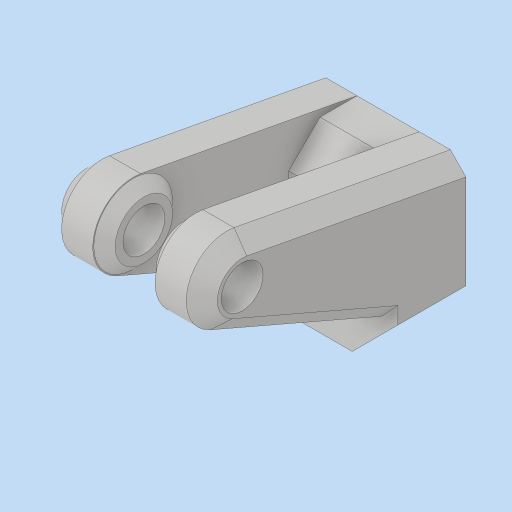
# Autodesk Inventor part: Profil-WheelHold-wBearing
Saved by Autodesk Inventor 2024 (Build 280153000, 153)
## iProperties
Created: 2023-04-19
Part Number: Profil-WheelHold-wBearing
Material: Generic
Document SubType Name: Modeling
Designer: Karbosch
Density: 1 g/cm^3
Appearance: Default
Mass: 3.2214 g
Surface Area: 21.1129 cm^2
Volume: 3.2214 cm^3
Author: Karbosch
Autodesk Inventor part; units mm, degrees
ref_plane "YZ Plane" through (0, 0, 0) normal (1, 0, 0) x (0, 1, 0)
ref_plane "XZ Plane" through (0, 0, 0) normal (0, 1, 0) x (-1, 0, 0)
ref_plane "XY Plane" through (0, 0, 0) normal (0, 0, 1) x (1, 0, 0)
sketch "Sketch1" plane through (0, 0, 0) normal (0, 0, 1) x (1, 0, 0)
  circle A0 centre (0, 0) radius 2.15
  line L0 (3.3137, 8) -> (8, 3.3137)
  line L1 (8, 3.3137) -> (8, -3.3137)
  line L2 (8, -3.3137) -> (3.3137, -8)
  line L3 (3.3137, -8) -> (-3.3137, -8)
  line L4 (-3.3137, -8) -> (-8, -3.3137)
  line L5 (-8, -3.3137) -> (-8, 3.3137)
  line L6 (-8, 3.3137) -> (-3.3137, 8)
  line L7 (-3.3137, 8) -> (3.3137, 8)
  dimension "d0" = 4.3
  dimension "d1" = 16
  constraints: 16 end point, 2 coincident, 1 centre point, 1 horizontal, 17 other
  measures "d0" diameter of A0
  measures "d1" distance between parallel lines of L3 L7
extrude "Extrusion1" add sketch "Sketch1" along normal blind 7
sketch "Sketch2" plane through (8, -3.3137, 0) normal (1, 0, 0) x (0, 0, -1)
  line L0 (0, 0) -> (-7, 0) projected
  line L1 (0, 6.6274) -> (0, 0) projected
  line L2 (0, 11.3137) -> (0, 6.6274) projected
  circle A0 centre (-23, 11.4137) radius 2.15
  circle A1 centre (-23, 11.4137) radius 4.15
  line L3 (0, 11.3137) -> (-7, 11.3137) projected
  line L4 (0, 11.3137) -> (-22.2335, 15.4923)
  line L5 (-7, 0) -> (-7, -4.6863) projected
  line L6 (-7, 0) -> (-24.6423, 7.6025)
  line L7 (-7, 1.1637) -> (-7, 5.4637) projected
  line L8 (-7, 3.3137) -> (-11, 3.3137)
  line L9 (-11, 3.3137) -> (-11, 7.0137)
  circle A2 centre (-23, 11.4137) radius 11
  circle A3 centre (-23, 11.4137) radius 8.1
  line L10 (5.8437, 3.3137) -> (-35.0625, 3.3137) projected
  point P0 (0, 3.3137)
  dimension "d4" = 4.3
  dimension "d6" = 2
  dimension "d17" = 4
  dimension "d18" = 3.7
  dimension "d19" = 22
  dimension "d33" = 16.2
  dimension "d34" = 16
  constraints: 8 end point, 4 centre point, 3 coincident, 3 tangent, 2 point on circle, 1 horizontal, 1 midpoint, 1 vertical
  measures "d4" diameter of A0
  measures "d6" radial gap between concentric circles of A1 A0
  measures "d17" distance of L8.start L8.end
  measures "d18" distance of L8.end L9.end
  measures "d19" diameter of A2
  measures "d33" diameter of A3
  measures "d34" horizontal distance of L3.end A0.centre
extrude "Extrusion2" add sketch "Sketch2" against normal blind 4.8 contours L0 L6 L10 L8 L1 | L10 L8 L6 A2 L4 L2 L1 | L6 A3 L4 A2 | L6 A1 L4 A3 | A1 picked at (-16.2916, 10.7819)
sketch "Sketch4" plane through (0, 0, 7) normal (0, 0, 1) x (1, 0, 0)
  circle A0 centre (0, 0) radius 3.7
  dimension "d14" = 7.4
  constraints: 1 centre point, 1 coincident
  measures "d14" diameter of A0
extrude "Extrusion4" cut sketch "Sketch4" along normal through all
chamfer "Chamfer2" distance 1.6 angle 45 3 edges at (8, 9.3118, 26.9691) (8, 0.4875, 15.8212) (8, 10.0893, 11.1167)
chamfer "Chamfer3" distance 3.2 angle 45 1 edges at (-0.0569, 8, 7)
sketch "Sketch5" plane through (3.2, -3.3137, 0) normal (-1, 0, 0) x (0, 0, 1)
  circle A0 centre (23, 11.4137) radius 2.15 projected
  arc A1 (24.0091, 9.0719) -> (22.529, 13.9198) centre (23, 11.4137) ccw projected
  circle A2 centre (23, 11.4137) radius 2.95
  point P0 (0, 3.3137)
  dimension "d26" = 0.8
  constraints: 1 centre point, 1 coincident
  measures "d26" radial gap between concentric circles of A0 A2
extrude "Extrusion5" add sketch "Sketch5" along normal blind 1.1
chamfer "Chamfer4" distance 1.1 angle 45 1 edges at (3.2, 8.1, 20.05)
mirror "Mirror2" about plane through (0, 0, 0) normal (1, 0, 0) of "Extrusion2", "Extrusion5", "Chamfer4", "Chamfer2"
body "Solid1"
